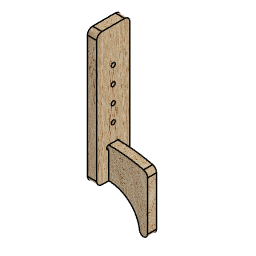
model (Autodesk Fusion 360 design; units mm, degrees)
Autodesk Fusion 360 part; units mm, degrees
sketch "Sketch1" plane through (0, 0, 0) normal (1, 0, 0) x (0, 1, 0)
  line L0 (0, 60) -> (64, 60)
  line L1 (64, 60) -> (64, 316.5)
  line L2 (64, 316.5) -> (0, 316.5)
  line L3 (0, 316.5) -> (0, 60)
  line L4 (0, 0) -> (0, 60) construction
  line L5 (32, 316.5) -> (32, 60) construction
  circle A0 centre (32, 153.5) radius 3.9688
  circle A1 centre (32, 185.5) radius 3.9688
  circle A2 centre (32, 217.5) radius 3.9688
  circle A3 centre (32, 249.5) radius 3.9688
  line L6 (23.25, 60) -> (23.25, 112.0625)
  arc A4 (23.25, 120) -> (23.25, 112.0625) centre (23.25, 116.0312) ccw
  line L7 (23.25, 120) -> (40.75, 120)
  line L8 (40.75, 60) -> (40.75, 112.0625)
  arc A5 (40.75, 112.0625) -> (40.75, 120) centre (40.75, 116.0312) ccw
  line L9 (40.75, 86.0312) -> (32, 86.0312) construction
  line L10 (32, 86.0312) -> (23.25, 86.0312) construction
  line L11 (23.25, 60) -> (23.25, 0)
  line L12 (23.25, 0) -> (40.75, 0)
  line L13 (40.75, 0) -> (40.75, 60)
  line L14 (40.75, 112.0625) -> (40.75, 120)
  line L15 (23.25, 112.0625) -> (23.25, 120)
  dimension "d1" = 32
  dimension "d2" = 7.9375
  dimension "d5" = 0
  dimension "d6" = 32
  dimension "d7" = 153.5
  dimension "d8" = 67
  dimension "d9" = 60
  dimension "d11" = 17.5
  dimension "d12" = 120
  dimension "d13" = 33.5
  constraint horizontal L0
  constraint vertical L1
  constraint horizontal L2
  constraint vertical L3
  constraint coincident L4.start origin
  constraint vertical L4
  constraint midpoint L2 L5.start
  constraint midpoint L0 L5.end
  constraint coincident L5 A0.centre
  constraint coincident L0 L6.start
  constraint coincident L0 L8.start
  constraint vertical L6
  constraint vertical L8
  constraint tangent L7 A5
  constraint tangent A4 L7
  constraint horizontal L7
  constraint equal A4 A5
  constraint equal A0 A4
  constraint midpoint L8 L9.start
  constraint coincident L5 L9.end
  constraint midpoint L6 L10.end
  constraint equal L9 L10
  constraint vertical L11
  constraint horizontal L12
  constraint vertical L13
  constraint equal L4 L11
  constraint vertical L15
  constraint vertical L14
  measures "d1" distance of L2.end L5.start
  measures "d2" diameter of A0
  measures "d7" vertical distance of L4.start A0.centre
  measures "d8" vertical distance of L2.end A3.centre
  measures "d9" distance of L0.start L4.start
  measures "d11" distance of L6.start L8.start
  measures "d12" vertical distance of L4.start A4.start
  measures "d13" vertical distance of A0.centre A4.start
extrude "Extrude1" add sketch "Sketch1" against normal blind 18 contours L0 L1 L2 L3 L6 A4 L7 L8 A5 makes body 1
extrude "Extrude2" add sketch "Sketch1" along normal blind 8 from surface at -18 contours L0 L6 L7 L8 L14 L15 | A4 L15 | A5 L14 bodies 1
extrude "Extrude3" add sketch "Sketch1" along normal blind 120 from surface at -10 separate body contours L0 L6 L7 L8 L14 L15 | L0 L11 L12 L13 makes body 2
sketch "Sketch2" plane through (0, 23.25, 0) normal (0, -1, 0) x (1, 0, 0)
  line L0 (-10, 120) -> (-10, 0)
  line L1 (-10, 0) -> (110, 0)
  line L2 (110, 0) -> (110, 120)
  line L3 (110, 120) -> (-10, 120)
  arc A0 (60, 0) -> (0, 60) centre (0, 0) ccw
  line L4 (0, 60) -> (-10, 60)
  line L5 (0, 60) -> (75, 60) construction
  line L6 (75, 0) -> (75, 110)
  arc A1 (75, 110) -> (0, 120) centre (0, -166.25) ccw
  arc A2 (59.6088, 6.8405) -> (75, 7.7208) centre (67.2792, 7.7208) ccw
  point P0 (0, 60)
  point P1 (0, 120)
  dimension "d24" = 50
  dimension "d25" = 15
  constraint coincident L1 A0.start
  constraint coincident P0 A0.end
  constraint coincident A0.centre origin
  constraint midpoint L0 L4.end
  constraint horizontal L5
  constraint coincident L1 L6.start
  constraint vertical L6
  constraint coincident L5.end L6
  constraint tangent L3 A1
  constraint coincident P1 A1.end
  constraint tangent L1 A2
  constraint coincident L6 A2.end
  constraint coincident A0 A2.start
  constraint tangent A0 A2
  constraint tangent L6 A2
  measures "d24" distance of L5.end L6.end
  measures "d25" distance of A0.start L6.start
extrude "Extrude4" cut sketch "Sketch2" against normal through all contours L0 L1 A0 L4 | L1 L2 L3 L6 A1 | L1 A0 A2 | L1 L6 A2 bodies 2
fillet "Fillet1" radius 10 5 edges at (-9, 0, 316.5) (-9, 64, 316.5) (-9, 0, 60) (-9, 64, 60) (75, 32, 110) on bodies 1 2
equation "d2 = 5/16\""
equation "d8 = d1 + 35 mm"
